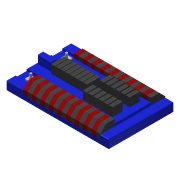
# Autodesk Inventor part: Power Distribution Board
Saved by Autodesk Inventor 2013 (Build 170138000, 138)
## iProperties
Created: 2013-12-22
Part Number: Power Distribution Board
Material: Generic
Document SubType Name: Modeling
Designer: Nemo
Density: 0.785451 g/cm^3
Mass: 725.748 g
Surface Area: 2067.06 cm^2
Volume: 923.988 cm^3
Author: Nemo
Autodesk Inventor part; units mm, degrees
ref_plane "YZ Plane" through (0, 0, 0) normal (1, 0, 0) x (0, 1, 0)
ref_plane "XZ Plane" through (0, 0, 0) normal (0, 1, 0) x (-1, 0, 0)
ref_plane "XY Plane" through (0, 0, 0) normal (0, 0, 1) x (1, 0, 0)
sketch "Sketch2" plane through (0, 0, 0) normal (0, 1, 0) x (-1, 0, 0)
  line L0 (0, 0) -> (228.6, 0)
  line L1 (228.6, 0) -> (228.6, 144.78)
  line L2 (228.6, 144.78) -> (0, 144.78)
  line L3 (0, 144.78) -> (0, 0)
  dimension "d0" = 228.6
  dimension "d2" = 144.78
  constraints: 8 end point, 2 parallel, 1 horizontal, 1 perpendicular
  measures "d0" distance between parallel lines of L1 L3
  measures "d2" distance of L2.end L0.start
extrude "Extrusion1" add sketch "Sketch2" along normal blind 9.652
sketch "Sketch3" plane through (0, 9.652, 0) normal (0, 1, 0) x (1, 0, 0)
  line L0 (0, 0) -> (-228.6, 0) construction
  line L1 (-228.6, -144.78) -> (0, -144.78) construction
  line L2 (0, -144.78) -> (0, 0) construction
  line L3 (-28.575, -113.03) -> (-19.05, -113.03)
  line L4 (-19.05, -113.03) -> (-19.05, -144.78)
  line L5 (-19.05, -144.78) -> (-28.575, -144.78)
  line L6 (-28.575, -144.78) -> (-28.575, -113.03)
  line L7 (-28.575, 0) -> (-19.05, 0)
  line L8 (-19.05, 0) -> (-19.05, -31.75)
  line L9 (-19.05, -31.75) -> (-28.575, -31.75)
  line L10 (-28.575, -31.75) -> (-28.575, 0)
  dimension "d5" = 19.05
  dimension "d6" = 31.75
  dimension "d14" = 9.525
  constraints: 16 end point, 5 collinear, 4 parallel, 2 horizontal, 2 perpendicular
  measures "d5" distance between parallel lines of L2 L4
  measures "d6" distance of L5.end L3.start
  measures "d14" distance of L3.start L3.end
extrude "Extrusion4" add sketch "Sketch3" along normal blind 24.13 separate body
sketch "Sketch5" plane through (0, 9.652, 0) normal (0, 1, 0) x (1, 0, 0)
  line L0 (0, 0) -> (-228.6, 0) projected
  line L1 (-228.6, -144.78) -> (0, -144.78) projected
  line L2 (-19.05, 0) -> (-28.575, 0) projected
  line L3 (-28.575, 0) -> (-28.575, -31.75) projected
  line L4 (-28.575, -31.75) -> (-19.05, -31.75) projected
  line L5 (-19.05, -31.75) -> (-19.05, 0) projected
  line L6 (-19.05, -113.03) -> (-28.575, -113.03) projected
  line L7 (-28.575, -113.03) -> (-28.575, -144.78) projected
  line L8 (-28.575, -144.78) -> (-19.05, -144.78) projected
  line L9 (-19.05, -144.78) -> (-19.05, -113.03) projected
  line L10 (-28.575, -31.75) -> (-38.1, -31.75)
  line L11 (-38.1, -31.75) -> (-38.1, 0)
  line L12 (-38.1, 0) -> (-28.575, 0)
  line L13 (-28.575, 0) -> (-28.575, -31.75)
  line L14 (-28.575, -113.03) -> (-38.1, -113.03)
  line L15 (-38.1, -113.03) -> (-38.1, -144.78)
  line L16 (-38.1, -144.78) -> (-28.575, -144.78)
  line L17 (-28.575, -144.78) -> (-28.575, -113.03)
  dimension "d19" = 9.525
  dimension "d20" = 9.525
  constraints: 16 end point, 4 parallel, 2 horizontal, 2 perpendicular, 2 point on line
  measures "d19" distance of L6.end L14.end
  measures "d20" distance of L3.end L10.end
extrude "Extrusion5" add sketch "Sketch5" along normal blind 24.13 separate body contours L3 L10 L11 L0 | L15 L14 L7 L1
pattern_linear "Rectangular Pattern2" count 9 spacing 19.05 along (-1, 0, 0) of "Extrusion4" bodies 2
pattern_linear "Rectangular Pattern3" count 9 spacing 19.05 along (-1, 0, 0) of "Extrusion5" bodies 3
sketch "Sketch6" plane through (0, 9.652, 0) normal (0, 1, 0) x (1, 0, 0)
  line L0 (-190.5, 0) -> (-190.5, -31.75) construction
  line L1 (-190.5, -31.75) -> (-180.975, -31.75) construction
  line L2 (-180.975, -31.75) -> (-180.975, 0) construction
  line L3 (-180.975, 0) -> (-190.5, 0) construction
  line L4 (-19.05, 0) -> (-28.575, 0) construction
  line L5 (-28.575, 0) -> (-28.575, -31.75) construction
  line L6 (-28.575, -31.75) -> (-19.05, -31.75) construction
  line L7 (-19.05, -31.75) -> (-19.05, 0) construction
  line L8 (-19.05, -113.03) -> (-28.575, -113.03) construction
  line L9 (-28.575, -113.03) -> (-28.575, -144.78) construction
  line L10 (-28.575, -144.78) -> (-19.05, -144.78) construction
  line L11 (-19.05, -144.78) -> (-19.05, -113.03) construction
  line L12 (-190.5, -144.78) -> (-180.975, -144.78) construction
  line L13 (-180.975, -144.78) -> (-180.975, -113.03) construction
  line L14 (-180.975, -113.03) -> (-190.5, -113.03) construction
  line L15 (-190.5, -113.03) -> (-190.5, -144.78) construction
  line L16 (-190.5, -113.03) -> (-19.05, -113.03)
  line L17 (-19.05, -113.03) -> (-19.05, -31.75)
  line L18 (-19.05, -31.75) -> (-190.5, -31.75)
  line L19 (-190.5, -31.75) -> (-190.5, -113.03)
  line L20 (-228.6, 0) -> (-190.5, 0)
  line L21 (-190.5, 0) -> (-190.5, -144.78)
  line L22 (-190.5, -144.78) -> (-228.6, -144.78)
  line L23 (-228.6, -144.78) -> (-228.6, 0)
  line L24 (-19.05, -144.78) -> (0, -144.78)
  line L25 (0, -144.78) -> (0, 0)
  line L26 (0, 0) -> (-19.05, 0)
  line L27 (-19.05, 0) -> (-19.05, -144.78)
  constraints: 24 end point, 6 parallel, 3 horizontal, 3 perpendicular
extrude "Extrusion6" add sketch "Sketch6" along normal blind 9.525 draft 0.375 bodies 1
sketch "Sketch7" plane through (0, 19.177, 0) normal (0, 1, 0) x (1, 0, 0)
  line L0 (-190.4377, -31.6877) -> (-19.1123, -31.6877)
  line L1 (-19.1123, -31.6877) -> (-19.1123, -113.0923)
  line L2 (-19.1123, -113.0923) -> (-190.4377, -113.0923)
  line L3 (-190.4377, -113.0923) -> (-190.4377, -31.6877)
  point P0 (0, 0)
  constraints: 8 end point, 2 parallel, 1 horizontal, 1 perpendicular
extrude "Extrusion7" add sketch "Sketch7" along normal blind 5.207 bodies 1
sketch "Sketch8" plane through (0, 19.177, 0) normal (0, 1, 0) x (1, 0, 0)
  line L0 (-228.6623, -144.8423) -> (-228.6623, 0.0623) projected
  line L1 (-225.069, -65.9684) -> (-194.245, -65.9684)
  line L2 (-194.245, -65.9684) -> (-194.245, -78.8116)
  line L3 (-194.245, -78.8116) -> (-225.069, -78.8116)
  line L4 (-225.069, -78.8116) -> (-225.069, -65.9684)
  point P0 (0, 0)
  point P1 (-225.069, -72.39)
  point P2 (-228.6623, -72.39)
  constraints: 8 end point, 2 midpoint, 2 parallel, 1 horizontal, 1 horizontal alignment, 1 perpendicular
extrude "Extrusion8" add sketch "Sketch8" along normal blind 19.05 bodies 1
fillet "Fillet1" radius 1.5875 33 edges at (-114.3, 0, 0) (0, 0, 72.39) (-114.3, 0, 144.78) (-228.6, 0, 72.39) (-209.657, 38.227, 65.9684) (-225.069, 38.227, 72.39) (-209.657, 38.227, 78.8116) (-194.245, 38.227, 72.39) (-225.069, 28.702, 65.9684) (-225.069, 28.702, 78.8116) (-228.6623, 19.177, 72.39) (-209.55, 19.177, -0.0623) (-209.55, 19.177, 144.8423) (-190.4377, 24.384, 72.39) (-228.6312, 14.4145, -0.0312) (-228.6, 4.826, 0) (-228.6, 4.826, 144.78) (-228.6312, 14.4145, 144.8112) (-194.245, 28.702, 78.8116) (-194.245, 28.702, 65.9684) (-209.657, 19.177, 65.9684) (-225.069, 19.177, 72.39) (-209.657, 19.177, 78.8116) (-194.245, 19.177, 72.39) (-19.1123, 24.384, 72.39) (-19.1123, 19.177, 72.39) (0.0623, 19.177, 72.39) (-9.525, 19.177, 144.8423) (-9.525, 19.177, -0.0623) (0.0312, 14.4145, -0.0312) (0, 4.826, 0) (0, 4.826, 144.78) (0.0312, 14.4145, 144.8112)
chamfer "Chamfer1" distance 12.7 angle 45 36 edges at (-23.8125, 33.782, 144.78) (-42.8625, 33.782, 144.78) (-61.9125, 33.782, 144.78) (-80.9625, 33.782, 144.78) (-100.0125, 33.782, 144.78) (-119.0625, 33.782, 144.78) (-138.1125, 33.782, 144.78) (-157.1625, 33.782, 144.78) (-176.2125, 33.782, 144.78) (-23.8125, 33.782, 0) (-42.8625, 33.782, 0) (-61.9125, 33.782, 0) (-80.9625, 33.782, 0) (-100.0125, 33.782, 0) (-119.0625, 33.782, 0) (-138.1125, 33.782, 0) (-157.1625, 33.782, 0) (-176.2125, 33.782, 0) (-33.3375, 33.782, 144.78) (-52.3875, 33.782, 144.78) (-71.4375, 33.782, 144.78) (-90.4875, 33.782, 144.78) (-109.5375, 33.782, 144.78) (-128.5875, 33.782, 144.78) (-147.6375, 33.782, 144.78) (-166.6875, 33.782, 144.78) (-185.7375, 33.782, 144.78) (-33.3375, 33.782, 0) (-52.3875, 33.782, 0) (-71.4375, 33.782, 0) (-90.4875, 33.782, 0) (-109.5375, 33.782, 0) (-128.5875, 33.782, 0) (-147.6375, 33.782, 0) (-166.6875, 33.782, 0) (-185.7375, 33.782, 0)
sketch "Sketch9" plane through (0, 24.384, 0) normal (0, 1, 0) x (1, 0, 0)
  line L0 (-188.8502, -113.0923) -> (-188.8502, -31.6877) construction
  line L1 (-186.3102, -57.785) -> (-177.4202, -57.785)
  line L2 (-177.4202, -57.785) -> (-177.4202, -86.995)
  line L3 (-177.4202, -86.995) -> (-186.3102, -86.995)
  line L4 (-186.3102, -86.995) -> (-186.3102, -57.785)
  point P0 (0, 0)
  point P1 (-186.3102, -72.39)
  point P2 (-188.8502, -72.39)
  dimension "d39" = 29.21
  dimension "d41" = 8.89
  dimension "d44" = 2.54
  constraints: 8 end point, 2 midpoint, 2 parallel, 1 horizontal, 1 horizontal alignment, 1 perpendicular
  measures "d39" distance of L3.end L1.start
  measures "d41" distance of L1.start L1.end
  measures "d44" distance between parallel lines of L4 L0
extrude "Extrusion9" add sketch "Sketch9" along normal blind 19.05 separate body
pattern_linear "Rectangular Pattern4" count 8 spacing 10.16 along (1, 0, 0) of "Extrusion9" bodies 4
sketch "Sketch10" plane through (0, 24.384, 0) normal (0, 1, 0) x (1, 0, 0)
  line L0 (-99.9502, -42.2275) -> (-91.0602, -42.2275)
  line L1 (-91.0602, -42.2275) -> (-91.0602, -64.4525)
  line L2 (-91.0602, -64.4525) -> (-99.9502, -64.4525)
  line L3 (-99.9502, -64.4525) -> (-99.9502, -42.2275)
  line L4 (-106.3002, -86.995) -> (-106.3002, -57.785) projected
  line L5 (-99.9502, -80.3275) -> (-91.0602, -80.3275)
  line L6 (-91.0602, -80.3275) -> (-91.0602, -102.5525)
  line L7 (-91.0602, -102.5525) -> (-99.9502, -102.5525)
  line L8 (-99.9502, -102.5525) -> (-99.9502, -80.3275)
  line L9 (-95.5052, -64.4525) -> (-95.5052, -80.3275) construction
  point P0 (0, 0)
  point P1 (-95.5052, -72.39)
  point P2 (-106.3002, -72.39)
  dimension "d48" = 8.89
  dimension "d49" = 22.225
  dimension "d50" = 6.35
  dimension "d51" = 8.89
  dimension "d52" = 22.225
  dimension "d53" = 15.875
  constraints: 18 end point, 4 midpoint, 4 parallel, 2 horizontal, 2 perpendicular, 1 horizontal alignment
  measures "d48" distance of L1.end L2.end
  measures "d49" distance of L2.end L0.start
  measures "d50" distance between parallel lines of L3 L4
  measures "d51" distance of L5.start L5.end
  measures "d52" distance of L7.end L5.start
  measures "d53" distance of L9.start L9.end
extrude "Extrusion10" add sketch "Sketch10" along normal blind 19.05 separate body
pattern_linear "Rectangular Pattern5" count 6 spacing 11.43 along (1, 0, 0) of "Extrusion10" bodies 5
sketch "Sketch11" plane through (0, 19.177, 0) normal (0, 1, 0) x (1, 0, 0)
  line L0 (-190.4377, -113.0923) -> (-190.4377, -31.6877) projected
  line L1 (-223.4815, -80.3991) -> (-195.8325, -80.3991) projected
  line L2 (-195.8325, -64.3809) -> (-223.4815, -64.3809) projected
  line L3 (-244.4127, -19.9309) -> (-199.9627, -19.9309)
  line L4 (-193.6127, -26.2809) -> (-193.6127, -38.9809)
  line L5 (-199.9627, -45.3309) -> (-244.4127, -45.3309)
  line L6 (-244.4127, -45.3309) -> (-244.4127, -19.9309)
  line L7 (-244.4127, -99.4491) -> (-199.9627, -99.4491)
  line L8 (-193.6127, -105.7991) -> (-193.6127, -118.4991)
  line L9 (-199.9627, -124.8491) -> (-244.4127, -124.8491)
  line L10 (-244.4127, -124.8491) -> (-244.4127, -99.4491)
  arc A0 (-193.6127, -26.2809) -> (-199.9627, -19.9309) centre (-199.9627, -26.2809) ccw
  arc A1 (-199.9627, -45.3309) -> (-193.6127, -38.9809) centre (-199.9627, -38.9809) ccw
  arc A2 (-193.6127, -105.7991) -> (-199.9627, -99.4491) centre (-199.9627, -105.7991) ccw
  arc A3 (-199.9627, -124.8491) -> (-193.6127, -118.4991) centre (-199.9627, -118.4991) ccw
  point P0 (0, 0)
  dimension "d59" = 25.4
  dimension "d61" = 3.175
  dimension "d62" = 50.8
  dimension "d63" = 19.05
  dimension "d64" = 19.05
  dimension "d65" = 6.35
  constraints: 16 end point, 8 point on circle, 8 tangent, 4 centre point, 4 parallel, 3 collinear, 3 equal radius, 2 horizontal, 2 perpendicular
  measures "d59" distance of L5.end L3.start
  measures "d61" distance between parallel lines of L0 L4
  measures "d62" distance between parallel lines of L4 L6
  measures "d63" distance between parallel lines of L7 L1
  measures "d64" distance between parallel lines of L2 L5
  measures "d65" radius of A0
extrude "Extrusion11" cut sketch "Sketch11" against normal blind 4.572 bodies 1
sketch "Sketch12" plane through (0, 14.605, 0) normal (0, 1, 0) x (1, 0, 0)
  line L0 (-228.6324, -45.3309) -> (-228.6324, -19.9309) construction
  line L1 (-193.6127, -26.2809) -> (-193.6127, -38.9809) construction
  line L2 (-212.7574, -26.1285) -> (-199.7526, -26.1285)
  line L3 (-199.7526, -26.1285) -> (-199.7526, -39.1333)
  line L4 (-199.7526, -39.1333) -> (-212.7574, -39.1333)
  line L5 (-212.7574, -39.1333) -> (-212.7574, -26.1285)
  point P0 (0, 0)
  point P1 (-199.7526, -32.6309)
  point P2 (-193.6127, -32.6309)
  dimension "d68" = 13.0048
  dimension "d70" = 13.0048
  dimension "d71" = 15.875
  constraints: 8 end point, 2 midpoint, 2 parallel, 1 horizontal, 1 horizontal alignment, 1 perpendicular
  measures "d68" distance of L2.start L2.end
  measures "d70" distance of L4.end L2.start
  measures "d71" distance between parallel lines of L0 L5
extrude "Extrusion12" add sketch "Sketch12" along normal blind 3.175 separate body
sketch "Sketch13" plane through (0, 17.78, 0) normal (0, 1, 0) x (1, 0, 0)
  circle A0 centre (-206.255, -32.6309) radius 2.5
  point P0 (0, 0)
  dimension "d74" = 5
  constraints: 1 centre point
  measures "d74" diameter of A0
extrude "Extrusion13" add sketch "Sketch13" along normal blind 10.16 bodies 6
pattern_linear "Rectangular Pattern6" count 2 spacing 79.5274 along (0, 0, 1) of "Extrusion12", "Extrusion13" bodies 6
move or copy body "Move Body1" bodies to move or copy 1 2 3 5 4 6 copy no translate (0, 0, -72.39)
body "Solid4"
body "Solid5"
body "Solid6"
body "Solid7"
body "Solid8"
